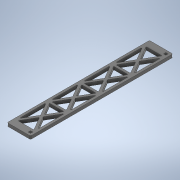
# Autodesk Inventor part: mount_battery_fastener
Saved by Autodesk Inventor 2022 (Build 260153000, 153)
## iProperties
Created: 2021-01-30
Part Number: mount_battery_fastener
Material: ABS Plastic
Document SubType Name: Modeling
Designer: User
Density: 1.06 g/cm^3
Appearance: Smooth - Black
Author: User
Autodesk Inventor part; units mm, degrees
ref_plane "YZ Plane" through (0, 0, 0) normal (1, 0, 0) x (0, 1, 0)
ref_plane "XZ Plane" through (0, 0, 0) normal (0, 1, 0) x (-1, 0, 0)
ref_plane "XY Plane" through (0, 0, 0) normal (0, 0, 1) x (1, 0, 0)
sketch "Sketch1" plane through (0, 0, 0) normal (0, 1, 0) x (-1, 0, 0)
  line L0 (-10, 0) -> (-10, 60)
  line L1 (-9, 61) -> (9, 61)
  line L2 (10, 60) -> (10, 0)
  line L3 (0, 0) -> (0, 61) construction
  arc A0 (-9, 61) -> (-10, 60) centre (-9, 60) ccw
  arc A1 (10, 60) -> (9, 61) centre (9, 60) ccw
  line L4 (10, 0) -> (-10, 0) construction
  line L5 (8, 55) -> (-8, 55)
  line L6 (8, 55) -> (8, 0)
  line L7 (-8, 55) -> (-8, 0)
  line L8 (8, 55) -> (-8, 27.5) construction
  line L9 (8, 0) -> (-8, 27.5) construction
  line L10 (-8, 0) -> (8, 27.5) construction
  line L11 (-8, 55) -> (8, 27.5) construction
  line L12 (-8, 27.5) -> (8, 27.5) construction
  line L13 (8, 1.9885) -> (1.1569, 13.75)
  line L14 (1.1569, 13.75) -> (8, 25.5115)
  line L15 (8, 29.4885) -> (1.1569, 41.25)
  line L16 (1.1569, 41.25) -> (8, 53.0115)
  line L17 (-1.1569, 41.25) -> (-8, 29.4885)
  line L18 (-1.1569, 41.25) -> (-8, 53.0115)
  line L19 (6.2612, 26.5) -> (0, 15.7385)
  line L20 (0, 15.7385) -> (-6.2612, 26.5)
  line L21 (-6.2612, 26.5) -> (6.2612, 26.5)
  line L22 (6.2612, 28.5) -> (-6.2612, 28.5)
  line L23 (-6.2612, 28.5) -> (0, 39.2615)
  line L24 (0, 39.2615) -> (6.2612, 28.5)
  line L25 (-1.1569, 13.75) -> (-8, 1.9885)
  line L26 (-1.1569, 13.75) -> (-8, 25.5115)
  line L27 (0, 43.2385) -> (6.8431, 55)
  line L28 (0, 43.2385) -> (-6.8431, 55)
  line L29 (6.2612, 1) -> (-6.2612, 1)
  line L30 (-6.2612, 1) -> (0, 11.7615)
  line L31 (6.2612, 1) -> (0, 11.7615)
  line L32 (-10, 0) -> (-10, -60)
  line L33 (-9, -61) -> (9, -61)
  line L34 (10, -60) -> (10, 0)
  arc A2 (-10, -60) -> (-9, -61) centre (-9, -60) ccw
  arc A3 (9, -61) -> (10, -60) centre (9, -60) ccw
  line L35 (8, -55) -> (-8, -55)
  line L36 (8, -55) -> (8, 0)
  line L37 (-8, -55) -> (-8, 0)
  line L38 (8, -55) -> (-8, -27.5) construction
  line L39 (8, 0) -> (-8, -27.5) construction
  line L40 (-8, 0) -> (8, -27.5) construction
  line L41 (-8, -55) -> (8, -27.5) construction
  line L42 (-8, -27.5) -> (8, -27.5) construction
  line L43 (8, -1.9885) -> (1.1569, -13.75)
  line L44 (1.1569, -13.75) -> (8, -25.5115)
  line L45 (8, -29.4885) -> (1.1569, -41.25)
  line L46 (1.1569, -41.25) -> (8, -53.0115)
  line L47 (-1.1569, -41.25) -> (-8, -29.4885)
  line L48 (-1.1569, -41.25) -> (-8, -53.0115)
  line L49 (6.2612, -26.5) -> (0, -15.7385)
  line L50 (0, -15.7385) -> (-6.2612, -26.5)
  line L51 (-6.2612, -26.5) -> (6.2612, -26.5)
  line L52 (6.2612, -28.5) -> (-6.2612, -28.5)
  line L53 (-6.2612, -28.5) -> (0, -39.2615)
  line L54 (0, -39.2615) -> (6.2612, -28.5)
  line L55 (-1.1569, -13.75) -> (-8, -1.9885)
  line L56 (-1.1569, -13.75) -> (-8, -25.5115)
  line L57 (0, -43.2385) -> (6.8431, -55)
  line L58 (0, -43.2385) -> (-6.8431, -55)
  line L59 (6.2612, -1) -> (-6.2612, -1)
  line L60 (-6.2612, -1) -> (0, -11.7615)
  line L61 (6.2612, -1) -> (0, -11.7615)
  line L62 (-8, 59) -> (-6, 59)
  line L63 (-6, 59) -> (-6, 57)
  line L64 (-6, 57) -> (-8, 57)
  line L65 (-8, 57) -> (-8, 59)
  line L66 (-8, 57) -> (-8, 55)
  line L67 (-8, 59) -> (-8, 61)
  line L68 (-8, -59) -> (-6, -59)
  line L69 (-6, -59) -> (-6, -57)
  line L70 (-6, -57) -> (-8, -57)
  line L71 (-8, -57) -> (-8, -59)
  point P0 (-10, 61)
  point P1 (10, 61)
  point P2 (0, 0)
  point P3 (-10, -61)
  point P4 (10, -61)
  point P5 (0, -61)
  dimension "d6" = 20
  dimension "d11" = 1
  dimension "d21" = 2
  dimension "d22" = 2
  dimension "d23" = 2
  dimension "d25" = 2
  dimension "d26" = 2
  dimension "d28" = 2
  dimension "d29" = 2
  dimension "d30" = 2
  dimension "d31" = 2
  dimension "d32" = 2
  dimension "d33" = 2
  dimension "d38" = 2
  dimension "d39" = 2
  dimension "d40" = 2
  dimension "d41" = 2
  dimension "d42" = 2
  dimension "d43" = 2
  dimension "d47" = 2
  dimension "d48" = 2
  dimension "d53" = 60
  dimension "d54" = 6
  constraints: 144 end point, 41 symmetric about line, 32 point on line, 19 parallel, 8 point on circle, 7 midpoint, 6 perpendicular, 5 horizontal, 4 centre point, 4 horizontal alignment, 4 tangent, 2 equal length, 2 vertical, 2 vertical alignment, 1 equal radius, 3 other
  measures "d6" distance of point (-10, 61) point (10, 61)
  measures "d11" radius of A0
  measures "d21" distance between parallel lines of L0 L7
  measures "d22" distance between parallel lines of L2 L6
  measures "d23" diameter of L13 L9
  measures "d25" diameter of L14 L10
  measures "d26" diameter of L19 L10
  measures "d28" diameter of L25 L10
  measures "d29" diameter of L21 L12
  measures "d30" diameter of L22 L12
  measures "d31" diameter of L24 L11
  measures "d32" diameter of L15 L11
  measures "d33" diameter of L16 L8
  measures "d38" diameter of L18 L11
  measures "d39" diameter of L17 L8
  measures "d40" diameter of L28 L11
  measures "d41" diameter of L26 L9
  measures "d42" diameter of L29 L4
  measures "d43" diameter of L31 L9
  measures "d47" distance of L64.end L62.start
  measures "d48" distance of L62.start L62.end
  measures "d53" distance of L0.start L32.end
  measures "d54" distance between parallel lines of L1 L5
extrude "Extrusion2" add sketch "Sketch1" along normal blind 2.6 contours L0 A0 L1 A1 L2 L34 A3 L33 A2 L32 | L6 L16 L15 L14 L13 L36 L43 L44 L45 L46 L35 L57 L58 L37 L48 L47 L56 L55 L7 L25 L26 L17 L18 L5 L28 L27 | L62 L63 L64 L65 | L71 L70 L69 L68
fillet "Fillet1" radius 0.4 47 edges at (-8, 1.3, 53.0115) (-8, 1.3, 29.4885) (-1.1569, 1.3, 41.25) (-6.8431, 1.3, 55) (0, 1.3, 43.2385) (6.8431, 1.3, 55) (8, 1.3, 53.0115) (1.1569, 1.3, 41.25) (0, 1.3, 39.2615) (6.2612, 1.3, 28.5) (8, 1.3, 29.4885) (6.2612, 1.3, 26.5) (-6.2612, 1.3, 26.5) (-8, 1.3, 25.5115) (0, 1.3, 15.7385) (-1.1569, 1.3, 13.75) (6.2612, 1.3, 1) (-6.2612, 1.3, 1) (-8, 1.3, 1.9885) (0, 1.3, 11.7615) (1.1569, 1.3, 13.75) (8, 1.3, 1.9885) (8, 1.3, 25.5115) (-6.2612, 1.3, -1) (0, 1.3, -11.7615) (6.2612, 1.3, -1) (8, 1.3, -1.9885) (1.1569, 1.3, -13.75) (-1.1569, 1.3, -13.75) (-8, 1.3, -1.9885) (-8, 1.3, -25.5115) (-6.2612, 1.3, -26.5) (6.2612, 1.3, -26.5) (0, 1.3, -15.7385) (8, 1.3, -25.5115) (-6.2612, 1.3, -28.5) (0, 1.3, -39.2615) (6.2612, 1.3, -28.5) (8, 1.3, -29.4885) (1.1569, 1.3, -41.25) (8, 1.3, -53.0115) (6.8431, 1.3, -55) (-6.8431, 1.3, -55) (0, 1.3, -43.2385) (-8, 1.3, -53.0115) (-8, 1.3, -29.4885) (-1.1569, 1.3, -41.25)
extrude "Extrusion3" cut sketch "Sketch1" along normal through all contours L62 L63 L64 L65 | L71 L70 L69 L68
equation "\"d21\" = link_width"
equation "\"d22\" = link_width"
equation "\"d23\" = link_width"
equation "\"d25\" = link_width"
equation "\"d26\" = link_width"
equation "\"d28\" = link_width"
equation "\"d29\" = link_width"
equation "\"d30\" = link_width"
equation "\"d31\" = link_width"
equation "\"d32\" = link_width"
equation "\"d33\" = link_width"
equation "\"d38\" = link_width"
equation "\"d39\" = link_width"
equation "\"d40\" = link_width"
equation "\"d41\" = link_width"
equation "\"d42\" = link_width"
equation "\"d43\" = link_width"
equation "\"link_width\" = 2"
body "Solid2"
